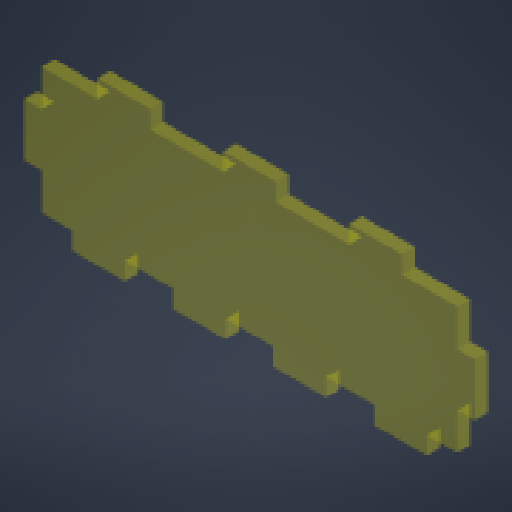
# Autodesk Inventor part: Acrilico-Parachoque
Saved by Autodesk Inventor 2026 (Build 300175000, 175)
## iProperties
Created: 2025-09-30
Part Number: Acrilico-Parachoque
Material: Genérico
Document SubType Name: Modeling
Designer: Nitro
Density: 1 g/cm^3
Appearance: Transparente - Amarelo
Author: Nitro
Autodesk Inventor part; units mm, degrees
ref_plane "YZ Plane" through (0, 0, 0) normal (1, 0, 0) x (0, 1, 0)
ref_plane "XZ Plane" through (0, 0, 0) normal (0, 1, 0) x (-1, 0, 0)
ref_plane "XY Plane" through (0, 0, 0) normal (0, 0, 1) x (1, 0, 0)
sketch "Esboço1" plane through (0, 0, 0) normal (0, 0, 1) x (1, 0, 0)
  line L0 (-59, 14.75) -> (43.5, 14.75)
  line L1 (43.5, 14.75) -> (43.5, -22)
  line L2 (43.5, -22) -> (-59, -22)
  line L3 (-59, -22) -> (-59, 14.75)
  point P0 (0, 0)
  dimension "d34" = 43.5
  dimension "d35" = 22
  dimension "d49" = 14.75
  dimension "d59" = 59
  constraints: 8 end point, 2 parallel, 1 horizontal, 1 perpendicular
  measures "d34" distance from line of L1 point (0, 0)
  measures "d35" distance from line of L2 point (0, 0)
  measures "d49" distance from line of point (0, 0) L0
  measures "d59" distance from line of L3 point (0, 0)
extrude "Extrusão1" add sketch "Esboço1" along normal blind 3
sketch "Esboço2" plane through (0, 0, 3) normal (0, 0, 1) x (1, 0, 0)
  line L0 (-59, -22) -> (43.5, -22) projected
  line L1 (43.5, -22) -> (42.5, -22)
  line L2 (43.5, 14.75) -> (26.875, 14.75)
  line L3 (26.875, 14.75) -> (26.875, 10.75)
  line L4 (26.875, 10.75) -> (43.5, 10.75)
  line L5 (43.5, 10.75) -> (43.5, 14.75)
  line L6 (14.875, 14.75) -> (-1.75, 14.75)
  line L7 (-1.75, 14.75) -> (-1.75, 10.75)
  line L8 (-1.75, 10.75) -> (14.875, 10.75)
  line L9 (14.875, 10.75) -> (14.875, 14.75)
  line L10 (-13.75, 14.75) -> (-30.375, 14.75)
  line L11 (-30.375, 14.75) -> (-30.375, 10.75)
  line L12 (-30.375, 10.75) -> (-13.75, 10.75)
  line L13 (-13.75, 10.75) -> (-13.75, 14.75)
  line L14 (-42.375, 14.75) -> (-59, 14.75)
  line L15 (-59, 14.75) -> (-59, 10.75)
  line L16 (-59, 10.75) -> (-42.375, 10.75)
  line L17 (-42.375, 10.75) -> (-42.375, 14.75)
  line L18 (43.5, -22) -> (32.6, -22)
  line L19 (32.6, -22) -> (32.6, -18)
  line L20 (32.6, -18) -> (43.5, -18)
  line L21 (43.5, -18) -> (43.5, -22)
  line L22 (9.7, -22) -> (9.7, -18)
  line L23 (20.6, -22) -> (19.6, -22)
  line L24 (20.6, -22) -> (9.7, -22)
  line L25 (20.6, -18) -> (20.6, -22)
  line L26 (9.7, -18) -> (20.6, -18)
  line L27 (-13.2, -22) -> (-13.2, -18)
  line L28 (-2.3, -22) -> (-3.3, -22)
  line L29 (-2.3, -22) -> (-13.2, -22)
  line L30 (-2.3, -18) -> (-2.3, -22)
  line L31 (-13.2, -18) -> (-2.3, -18)
  line L32 (-36.1, -22) -> (-36.1, -18)
  line L33 (-25.2, -22) -> (-26.2, -22)
  line L34 (-25.2, -22) -> (-36.1, -22)
  line L35 (-25.2, -18) -> (-25.2, -22)
  line L36 (-36.1, -18) -> (-25.2, -18)
  line L37 (-59, -22) -> (-59, -18)
  line L38 (-48.1, -22) -> (-49.1, -22)
  line L39 (-48.1, -22) -> (-59, -22)
  line L40 (-48.1, -18) -> (-48.1, -22)
  line L41 (-59, -18) -> (-48.1, -18)
  line L42 (-59, 14.75) -> (-59, -22) projected
  line L43 (-59, -22) -> (-59, -22)
  line L44 (-59, -22) -> (-59, -18)
  line L45 (-59, -18) -> (-59, -18)
  line L46 (-59, -18) -> (-59, -22)
  line L47 (-59, 10.75) -> (-59, 10.75)
  line L48 (-59, 10.75) -> (-59, 14.75)
  line L49 (-59, 14.75) -> (-59, 14.75)
  line L50 (-59, 14.75) -> (-59, 10.75)
  line L51 (-59, -18) -> (-59, -9.625) construction
  line L52 (-59, -9.625) -> (-55, -9.625) construction
  line L53 (-55, 2.375) -> (-59, 2.375) construction
  line L54 (-59, 2.375) -> (-59, -9.625) construction
  line L55 (-13.75, 14.75) -> (-13.75, -22) construction
  line L56 (43.5, -22) -> (43.5, 14.75) projected
  line L57 (43.5, -9.625) -> (39.5, -9.625) construction
  line L58 (39.5, 2.375) -> (43.5, 2.375) construction
  line L59 (43.5, 2.375) -> (43.5, -9.625)
  line L60 (39.5, -9.625) -> (43.5, -9.625)
  line L61 (43.5, -9.625) -> (43.5, -18)
  line L62 (43.5, -18) -> (39.5, -18)
  line L63 (39.5, -18) -> (39.5, -9.625)
  line L64 (39.5, 2.375) -> (43.5, 2.375)
  line L65 (43.5, 2.375) -> (43.5, 10.75)
  line L66 (43.5, 10.75) -> (39.5, 10.75)
  line L67 (39.5, 10.75) -> (39.5, 2.375)
  line L68 (-55, -9.625) -> (-59, -9.625)
  line L69 (-59, -9.625) -> (-59, -18)
  line L70 (-59, -18) -> (-55, -18)
  line L71 (-55, -18) -> (-55, -9.625)
  line L72 (-55, 2.375) -> (-59, 2.375)
  line L73 (-59, 2.375) -> (-59, 10.75)
  line L74 (-59, 10.75) -> (-55, 10.75)
  line L75 (-55, 10.75) -> (-55, 2.375)
  point P0 (-48.1, -22)
  point P1 (-36.1, -22)
  point P2 (-25.2, -22)
  point P3 (-13.2, -22)
  point P4 (-2.3, -22)
  point P5 (9.7, -22)
  point P6 (32.6, -22)
  point P7 (-57.4, -18)
  point P8 (-57, 14.75)
  dimension "d40" = 4
  dimension "d41" = 16.625
  dimension "d44" = 28.625
  dimension "d50" = 10.9
  dimension "d51" = 4
  dimension "d54" = 22.9
  dimension "d60" = 8.375
  constraints: 146 end point, 18 equal length, 12 horizontal, 9 perpendicular, 4 point on line, 64 other
  measures "d40" distance of L2.end L3.end
  measures "d41" distance of L3.end L4.end
  measures "d44" distance of L2.start L6.start
  measures "d50" distance of L19.end L20.end
  measures "d51" distance of L18.end L19.end
  measures "d54" distance of L19.end L22.end
  measures "d60" distance of L44.end L51.end
extrude "Extrusão2" cut sketch "Esboço2" against normal through all
